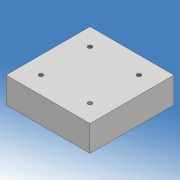
# Autodesk Inventor part: soporte_iman
Saved by Autodesk Inventor 2018.3 (Build 223284000, 284)
## iProperties
Created: 2019-03-20
Part Number: soporte_iman
Material: Generic
Document SubType Name: Modeling
Designer: vigus
Density: 1 g/cm^3
Appearance: Default
Author: vigus
Autodesk Inventor part; units mm, degrees
ref_plane "YZ Plane" through (0, 0, 0) normal (1, 0, 0) x (0, 1, 0)
ref_plane "XZ Plane" through (0, 0, 0) normal (0, 1, 0) x (-1, 0, 0)
ref_plane "XY Plane" through (0, 0, 0) normal (0, 0, 1) x (1, 0, 0)
sketch "Sketch1" plane through (0, 0, 0) normal (0, 0, 1) x (1, 0, 0)
  circle A0 centre (-17.5, -17.5) radius 1.5
  circle A1 centre (17.5, -17.5) radius 1.5
  circle A2 centre (17.5, 17.5) radius 1.5
  circle A3 centre (-17.5, 17.5) radius 1.5
  line L0 (-22.5, 22.5) -> (22.5, 22.5)
  line L1 (22.5, 22.5) -> (22.5, -22.5)
  line L2 (22.5, -22.5) -> (-22.5, -22.5)
  line L3 (-22.5, -22.5) -> (-22.5, 22.5)
  point P0 (0, 0)
  dimension "d4" = 3
  dimension "d5" = 3
  dimension "d6" = 3
  dimension "d7" = 3
  dimension "d8" = 35
  dimension "d9" = 35
  dimension "d10" = 35
  dimension "d13" = 45
  dimension "d14" = 45
  dimension "d15" = 22.5
  dimension "d16" = 22.5
  dimension "d17" = 5
  dimension "d18" = 5
  constraints: 8 end point, 4 centre point, 2 parallel, 1 horizontal, 1 perpendicular
  measures "d4" diameter of A0
  measures "d5" diameter of A1
  measures "d6" diameter of A2
  measures "d7" diameter of A3
  measures "d8" distance of A1.centre A2.centre
  measures "d9" distance of A0.centre A3.centre
  measures "d10" distance of A2.centre A3.centre
  measures "d13" distance of L1.end L2.end
  measures "d14" distance of L0.end L1.end
  measures "d15" distance from line of point (0, 0) L3
  measures "d16" distance from line of point (0, 0) L0
  measures "d17" distance from line of L3 A3.centre
  measures "d18" distance from line of L0 A3.centre
sketch "Sketch2" plane through (0, 0, 0) normal (0, 0, 1) x (1, 0, 0)
  line L0 (-30, 30) -> (30, 30)
  line L1 (30, 30) -> (30, -30)
  line L2 (30, -30) -> (-30, -30)
  line L3 (-30, -30) -> (-30, 30)
  point P0 (0, 0)
  dimension "d20" = 60
  dimension "d21" = 60
  dimension "d22" = 30
  dimension "d23" = 30
  constraints: 8 end point, 2 parallel, 1 horizontal, 1 perpendicular
  measures "d20" distance of L1.end L2.end
  measures "d21" distance of L0.end L1.end
  measures "d22" distance from line of point (0, 0) L0
  measures "d23" distance from line of point (0, 0) L3
extrude "Extrusion1" add sketch "Sketch2" along normal blind 18.5
extrude "Extrusion2" cut sketch "Sketch1" along normal blind 18
sketch "Sketch3" plane through (-17.5, 17.5, 0) normal (0, 0, -1) x (-1, 0, 0)
  circle A0 centre (0, 0) radius 1.5 projected
  circle A1 centre (0, -35) radius 1.5 projected
  circle A2 centre (-35, 0) radius 1.5 projected
  circle A3 centre (-35, -35) radius 1.5 projected
  point P0 (-17.5, -17.5)
extrude "Extrusion3" cut sketch "Sketch3" against normal blind 19
body "Solid1"
